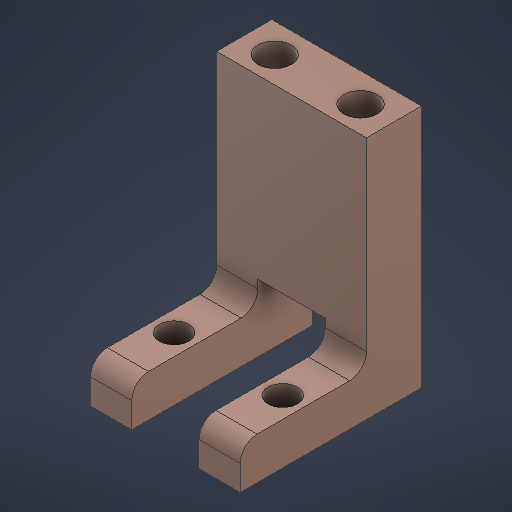
# Autodesk Inventor part: Sujeción de servo a mesa
Saved by Autodesk Inventor 2026 (Build 300175000, 175)
## iProperties
Created: 2025-08-24
Part Number: Sujeción de servo a mesa
Material: Plástico PC/ABS
Document SubType Name: Modeling
Designer: Thomas
Density: 1.1 g/cm^3
Appearance: Suave - Blanco
Author: Thomas
Autodesk Inventor part; units mm, degrees
ref_plane "YZ Plane" through (0, 0, 0) normal (1, 0, 0) x (0, 1, 0)
ref_plane "XZ Plane" through (0, 0, 0) normal (0, 1, 0) x (-1, 0, 0)
ref_plane "XY Plane" through (0, 0, 0) normal (0, 0, 1) x (1, 0, 0)
sketch "Boceto1" plane through (0, 0, 0) normal (1, 0, 0) x (0, 1, 0)
  line L0 (27, 0) -> (0, 0)
  line L1 (0, 0) -> (0, 6.55)
  line L2 (0, 6.55) -> (27, 6.55)
  line L3 (27, 6.55) -> (27, 0)
  line L4 (0, 6.55) -> (5, 6.55)
  line L5 (5, 6.55) -> (5, 21.55)
  line L6 (5, 21.55) -> (0, 21.55)
  line L7 (0, 21.55) -> (0, 6.55)
  dimension "d0" = 27
  dimension "d1" = 6.55
  dimension "d2" = 15
  dimension "d3" = 5
  constraints: 16 end point, 4 parallel, 2 horizontal, 2 perpendicular, 1 coincident
  measures "d0" distance of L0.start L0.end
  measures "d1" distance of L2.end L0.start
  measures "d2" distance of L4.end L5.end
  measures "d3" distance of L5.end L6.end
extrude "Extrusión1" add sketch "Boceto1" along normal mid plane 17.8
sketch "Boceto3" plane through (8.9, 27, 0) normal (0, 0, -1) x (-1, 0, 0)
  line L0 (4.9, -19) -> (12.9, -19)
  line L1 (12.9, -19) -> (12.9, -27)
  line L2 (12.9, -27) -> (4.9, -27)
  line L3 (4.9, -27) -> (4.9, -19)
  line L4 (0, -27) -> (17.8, -27) projected
  point P0 (8.9, -27)
  point P1 (8.9, -27)
  dimension "d6" = 8
  dimension "d7" = 8
  constraints: 8 end point, 2 midpoint, 2 parallel, 1 horizontal, 1 perpendicular
  measures "d6" distance of L1.end L2.end
  measures "d7" distance of L0.end L1.end
extrude "Extrusión2" cut sketch "Boceto3" against normal through all
sketch "Boceto4" plane through (-8.9, 5, 21.55) normal (0, 1, 0) x (1, 0, 0)
  point P0 (8.9, 21.55)
sketch "Boceto5" plane through (-8.9, 27, 6.55) normal (0, 1, 0) x (1, 0, 0)
  circle A0 centre (3.8, 3.1) radius 2
  circle A1 centre (14, 3.1) radius 2
  line L0 (0, 0) -> (0, 6.55) projected
  line L1 (0, 0) -> (17.8, 0) projected
  line L2 (17.8, 6.55) -> (17.8, 0) projected
  point P0 (8.9, 6.55)
  dimension "d10" = 4
  dimension "d11" = 4
  dimension "d12" = 3.8
  dimension "d13" = 3.1
  dimension "d14" = 3.8
  constraints: 2 centre point, 1 horizontal alignment
  measures "d10" diameter of A0
  measures "d11" diameter of A1
  measures "d12" distance from line of A0.centre L0
  measures "d13" distance from line of L1 A0.centre
  measures "d14" distance from line of L2 A1.centre
extrude "Extrusión3" cut sketch "Boceto5" against normal blind 10
sketch "Boceto6" plane through (-8.9, 5, 21.55) normal (0, 1, 0) x (1, 0, 0)
  circle A0 centre (2.45, 7.5) radius 1.75
  circle A1 centre (15.35, 7.5) radius 1.75
  line L0 (0, 0) -> (4.9, 0) projected
  line L1 (0, 15) -> (17.8, 15) projected
  line L2 (12.9, 0) -> (17.8, 0) projected
  point P0 (8.9, 21.55)
  point P1 (2.45, 0)
  point P2 (15.35, 0)
  dimension "d17" = 3.5
  dimension "d18" = 3.5
  dimension "d19" = 15
  dimension "d20" = 7.5
  dimension "d21" = 7.5
  constraints: 2 centre point, 2 midpoint, 2 vertical alignment
  measures "d17" diameter of A0
  measures "d18" diameter of A1
  measures "d19" distance from line of point (2.45, 0) L1
  measures "d20" distance from line of A0.centre L0
  measures "d21" distance from line of A1.centre L2
extrude "Extrusión4" cut sketch "Boceto6" against normal through all
fillet "Empalme1" radius 2 2 edges at (-6.45, 5, 6.55) (6.45, 5, 6.55)
fillet "Empalme2" radius 2 2 edges at (-6.45, 5, 21.55) (6.45, 5, 21.55)
move faces "Desplazar1" translate (0, 2, 0) faces at (1.6196, 27, 0.4882)
equation "\"d11\" = d10"
equation "\"d14\" = d12"
equation "\"d20\" = 0.5 * d19"
equation "\"d21\" = d20"
